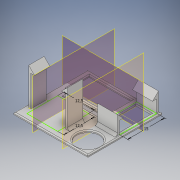
# Autodesk Inventor part: clip_12_5
Saved by Autodesk Inventor 2019 (Build 230136000, 136)
## iProperties
Created: 2019-01-17
Part Number: clip_12_5
Material: Generic
Document SubType Name: Modeling
Designer: assman
Density: 1 g/cm^3
Appearance: Default
Author: assman
Autodesk Inventor part; units mm, degrees
ref_plane "YZ Plane" through (0, 0, 0) normal (1, 0, 0) x (0, 1, 0)
ref_plane "XZ Plane" through (0, 0, 0) normal (0, 1, 0) x (-1, 0, 0)
ref_plane "XY Plane" through (0, 0, 0) normal (0, 0, 1) x (1, 0, 0)
sketch "Sketch1" plane through (0, 0, 0) normal (0, 0, 1) x (1, 0, 0)
  line L0 (0, 0) -> (-0.8, 0)
  line L1 (0, 0) -> (0, 12.5)
  line L2 (0, 12.5) -> (1.6, 12.5)
  line L3 (1.6, 12.5) -> (-0.8, 14.9)
  line L4 (-0.8, 14.9) -> (-0.8, 0)
  dimension "d1" = 0.8
  dimension "d2" = 12.5
  dimension "d3" = 1.6
  dimension "d4" = 45
  constraints: 10 end point, 2 horizontal, 1 perpendicular, 1 vertical
  measures "d1" distance of L0.start L0.end
  measures "d2" distance of L0.start L1.end
  measures "d3" distance of L1.end L2.end
  measures "d4" angle of L4 L3
extrude "Extrusion1" add sketch "Sketch1" along normal blind 6.25
sketch "Sketch2" plane through (-0.8, 0, 0) normal (0, -1, 0) x (1, 0, 0)
  line L0 (-1.4152, 10.8692) -> (28.5848, 10.8692)
  line L1 (28.5848, 10.8692) -> (28.5848, -19.1308)
  line L2 (28.5848, -19.1308) -> (-1.4152, -19.1308)
  line L3 (-1.4152, -19.1308) -> (-1.4152, 10.8692)
  point P0 (0.8, 0)
  dimension "d7" = 30
  dimension "d8" = 30
  dimension "d9" = 30
  constraints: 8 end point, 2 parallel, 1 horizontal, 1 perpendicular
  measures "d7" distance of L0.start L0.end
  measures "d8" distance of L1.end L2.end
  measures "d9" distance of L2.end L0.start
extrude "Extrusion2" add sketch "Sketch2" along normal blind 0.8 separate body
sketch "Sketch3" plane through (-0.8, 0, 0) normal (0, 1, 0) x (1, 0, 0)
  line L0 (0, -6.25) -> (0.8, -6.25) projected
  point P0 (0.8, 0)
sketch "Sketch4" plane through (-0.8, 0, 0) normal (0, 1, 0) x (1, 0, 0)
  line L0 (1.6, -8.662) -> (14.1, -8.662)
  line L1 (14.1, -8.662) -> (14.1, 3.838)
  line L2 (14.1, 3.838) -> (1.6, 3.838)
  line L3 (1.6, 3.838) -> (1.6, -8.662)
  line L4 (7.85, -8.662) -> (7.85, 3.838) construction
  point P0 (1.6, 0)
  dimension "d14" = 12.5
  dimension "d15" = 12.5
  constraints: 10 end point, 2 midpoint, 2 parallel, 1 horizontal, 1 perpendicular
  measures "d14" distance of L2.end L1.end
  measures "d15" distance of L1.end L0.end
ref_plane "Work Plane1" through (7.05, 0, 8.662) normal (1, 0, 0) x (0, 0, -1)
mirror "Mirror1" about plane through (7.05, 0, 8.662) normal (1, 0, 0) of "Extrusion1" bodies 1
sketch "Sketch5" plane through (0, 0, 0) normal (1, 0, 0) x (0, 1, 0)
  line L0 (0, -19.1308) -> (0, 10.8692) projected
  line L1 (0, -3.3308) -> (0, -4.1308)
  line L2 (0, 0) -> (14.9, 0) construction
  line L3 (0, -17.6889) -> (5, -17.6889)
  line L4 (5, -17.6889) -> (5, -16.0889)
  line L5 (5, -16.0889) -> (7.4, -18.4889)
  line L6 (7.4, -18.4889) -> (0, -18.4889)
  dimension "d24" = 5
  dimension "d25" = 1.6
  dimension "d26" = 0.8
  dimension "d27" = 45
  constraints: 10 end point, 2 perpendicular, 2 point on line, 1 horizontal, 1 midpoint
  measures "d24" distance of L3.start L3.end
  measures "d25" distance of L3.end L4.end
  measures "d26" distance between parallel lines of L3 L6
  measures "d27" angle of L6 L5
extrude "Extrusion3" add sketch "Sketch5" along normal blind 27 separate body
sketch "Sketch6" plane through (-0.8, 0, 0) normal (0, 1, 0) x (1, 0, 0)
  line L0 (19.7191, 17.6889) -> (27.7865, 17.6889)
  line L1 (27.7865, 17.6889) -> (27.7865, 2.6889)
  line L2 (27.7865, 2.6889) -> (19.7191, 2.6889)
  line L3 (19.7191, 2.6889) -> (19.7191, 17.6889)
  line L4 (19.7191, 10.1889) -> (27.7865, 10.1889) construction
  point P0 (0.8, 0)
  dimension "d28" = 15
  constraints: 10 end point, 2 midpoint, 2 parallel, 1 horizontal, 1 perpendicular
  measures "d28" distance of L0.end L1.end
ref_plane "Work Plane3" through (18.9191, 0, -2.6889) normal (1, 0, 0) x (0, 0, -1)
split "Split1" plane through (18.9191, 0, -2.6889) removes the side toward (-1, 0, 0) bodies 3
ref_plane "Work Plane4" through (18.9191, 0, -10.1889) normal (0, 0, 1) x (1, 0, 0)
mirror "Mirror2" about plane through (18.9191, 0, -10.1889) normal (0, 0, 1) of "Extrusion3" bodies 3
split "Split2" plane through (18.9191, 0, -2.6889) removes the side toward (-1, 0, 0) bodies 3
combine bodies "Combine1" operation type add bodies to combine 3 2
fillet "Fillet1" radius 1 1 edges at (22.9595, 0, -1.8889)
combine bodies "Combine2" operation type add bodies to combine 1 3
fillet "Fillet2" radius 1 1 edges at (14.9, 0, 3.125)
sketch "Sketch7" plane through (-2.2152, 0, 10.8692) normal (0, 1, 0) x (1, 0, 0)
  circle A0 centre (24.5881, 5.4446) radius 4.5779
  line L0 (2.2152, 19.1731) -> (19.416, 19.1731)
  line L1 (19.416, 19.1731) -> (19.416, 28.3041)
  line L2 (19.416, 28.3041) -> (2.2152, 28.3041)
  line L3 (2.2152, 28.3041) -> (2.2152, 19.1731)
  point P0 (2.2152, 10.8692)
  constraints: 8 end point, 2 parallel, 1 centre point, 1 horizontal, 1 perpendicular
extrude "Extrusion4" cut sketch "Sketch7" against normal blind 20 bodies 1
sketch "Sketch8" plane through (-2.2152, 0, 10.8692) normal (0, 1, 0) x (1, 0, 0)
  line L0 (21.6549, 13.9424) -> (28.4444, 13.9424)
  line L1 (28.4444, 13.9424) -> (28.4444, 27.736)
  line L2 (28.4444, 27.736) -> (21.6549, 27.736)
  line L3 (21.6549, 27.736) -> (21.6549, 13.9424)
  point P0 (2.2152, 10.8692)
  constraints: 8 end point, 2 parallel, 1 horizontal, 1 perpendicular
extrude "Extrusion5" cut sketch "Sketch8" against normal blind 20 bodies 1
sketch "Sketch9" plane through (-2.2152, 0, 10.8692) normal (0, 1, 0) x (1, 0, 0)
  line L0 (4.5196, 15.8107) -> (20.2749, 15.8107)
  line L1 (20.2749, 15.8107) -> (20.2749, 17.5612)
  line L2 (20.2749, 17.5612) -> (4.5196, 17.5612)
  line L3 (4.5196, 17.5612) -> (4.5196, 15.8107)
  point P0 (2.2152, 10.8692)
  constraints: 8 end point, 2 parallel, 1 horizontal, 1 perpendicular
extrude "Extrusion6" cut sketch "Sketch9" against normal blind 20 bodies 1
fillet "Fillet3" radius 0.4 13 edges at (12.7848, 0, 10.8692) (27.7848, 0, -4.1308) (12.7848, 0, -19.1308) (-2.2152, 0, -4.1308) (17.2008, 0, -12.8693) (8.6004, 0, -8.3038) (0, 0, -12.8693) (8.6004, 0, -17.4348) (17.795, 0, 5.4246) (18.0596, 0, -5.8167) (10.182, 0, -4.9414) (2.3044, 0, -5.8167) (10.182, 0, -6.692)
ref_plane "Work Plane2" through (7.05, 0, 8.662) normal (1, 0, 0) x (0, 0, -1)
ref_plane "Work Plane5" through (18.9191, 0, -10.1889) normal (0, 0, 1) x (1, 0, 0)
body "Solid2"
